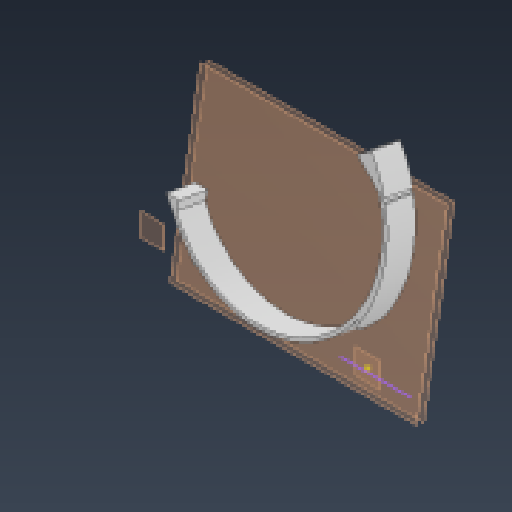
# Autodesk Inventor part: thigh_strap_03
Saved by Autodesk Inventor 2025.2 (Build 292293000, 293)
## iProperties
Created: 2025-03-07
Part Number: thigh_strap_03
Material: Generic
Document SubType Name: Modeling
Designer: email
Density: 1 g/cm^3
Appearance: Default
Author: email
Autodesk Inventor part; units mm, degrees
ref_plane "YZ Plane" through (0, 0, 0) normal (1, 0, 0) x (0, 1, 0)
ref_plane "XZ Plane" through (0, 0, 0) normal (0, 1, 0) x (-1, 0, 0)
ref_plane "Work Plane1" through (27.2016, 137.7902, -207.6153) normal (0, 0, 1) x (1, 0, 0)
ref_plane "Work Plane2" through (-81.5141, 115.844, -101.5145) normal (0, 0, 1) x (1, 0, 0)
sketch "Sketch2" plane through (27.2016, 137.7902, -207.6153) normal (0, 0, 1) x (1, 0, 0)
  line L0 (-50.9279, -141.1381) -> (10.2073, -141.1381)
  point P0 (-27.2016, -137.7902)
  constraints: 2 end point, 1 horizontal
ref_plane "Work Plane4" through (-23.7263, -2.2452, -201.3618) normal (0, 0.1736482, 0.9848078) x (1, 0, 0)
ref_plane "Work Plane3" through (-23.7263, -3.3479, -207.6153) normal (0, 0.1736482, 0.9848078) x (1, 0, 0)
sketch "Sketch1" plane through (-81.5141, 95.2083, -218.5455) normal (0, 0.1736482, 0.9848078) x (1, 0, 0)
  line L0 (120.3524, 26.6103) -> (110.8538, 39.0511) projected
  line L1 (109.9403, 39.2699) -> (118.8077, 27.6558) projected
  line L2 (117.4827, 25.3957) -> (118.8077, 27.6558) projected
  line L3 (108.6153, 37.0098) -> (109.9403, 39.2699) projected
  line L4 (-70.1644, -17.8234) -> (-70.1644, -42.3865) projected
  line L5 (-67.5144, -23.0328) -> (-67.5144, -49.6797) projected
  line L6 (-7.2549, -88.8185) -> (-7.2549, -90.7022)
  line L7 (88.6474, -22.0445) -> (90.1001, -24.6815)
  arc A0 (90.1001, -24.6815) -> (85.4909, 74.1551) centre (-2.6058, 20.521) ccw
  line L8 (68.6883, 59.486) -> (92.8567, 47.8109)
  ellipse E0 centre (117.3159, 24.5297) end of major axis (77.6327, 47.7943) minor radius 6.9177 (109.5288, 36.791) -> (89.1504, 46.193) ccw projected
  ellipse E1 centre (118.6409, 26.7898) end of major axis (80.226, 49.3108) minor radius 6.6966 (109.9403, 39.2699) -> (91.8991, 47.566) ccw projected
  line L9 (120.3524, 26.6103) -> (110.8538, 39.0511) projected
  line L10 (120.3524, 26.6103) -> (110.8538, 39.0511) projected
  line L11 (-70.1644, -47.9895) -> (-70.1644, -41.1809) projected
  line L12 (-78.1686, -54.9211) -> (-78.1686, -34.8) projected
  line L13 (-78.1686, -34.8) -> (-78.1686, -33.261) projected
  ellipse E2 centre (-68.1686, -34.8) end of major axis (-78.1686, -34.8) minor radius 8.1116 (-75.6686, -29.4347) -> (-78.1686, -34.8) ccw projected
  line L14 (-78.1686, -54.9211) -> (-78.1686, -34.8) projected
  line L15 (-77.6379, -18.1276) -> (-66.4488, -18.1276)
  line L16 (-66.4488, -18.1276) -> (-58.9889, -34.0305)
  arc A1 (-77.6379, -18.1276) -> (-51.8229, -55.9602) centre (98.8915, 74.6035) ccw
  line L17 (-51.8229, -55.9602) -> (-49.6664, -53.6662)
  ellipse E3 centre (43.7773, 28.2672) end of major axis (9.3333, 77.3077) minor radius 54.627 (86.8491, 61.886) -> (73.2137, 75.1203) ccw projected
  ellipse E4 centre (87.3016, 57.9812) end of major axis (48.0133, 78.9413) minor radius 0.2829 (58.2062, 73.2871) -> (75.8706, 63.7724) ccw projected
  ellipse E5 centre (86.0543, 55.6432) end of major axis (46.766, 76.6033) minor radius 0.2829 (56.9589, 70.9491) -> (74.6233, 61.4344) ccw projected
  ellipse E6 centre (-82.1686, -42.8548) end of major axis (-78.1686, -42.8548) minor radius 0.6946 (-78.1686, -42.8548) -> (-82.1686, -42.1602) ccw projected
  line L18 (85.4909, 74.1551) -> (63.6157, 67.3502)
  arc A2 (-66.1246, -22.0445) -> (76.0856, 61.886) centre (8.3655, 14.1852) ccw
  arc A3 (-70.1644, -30.1049) -> (79.8851, 69.6106) centre (7.0855, 16.4044) ccw
  line L19 (63.6157, 67.3502) -> (68.6883, 59.486)
  point P0 (81.5141, -131.7119)
  point P1 (-70.1644, -31.1405)
  point P2 (97.5203, 45.2683)
  point P3 (-67.5144, -35.2635)
  point P4 (96.3482, 45.7746)
  point P5 (98.1827, 42.4146)
  point P6 (110.3672, 38.7108)
  point P7 (-70.1644, -18.1276)
  point P8 (81.3429, 53.3729)
  point P9 (-67.5144, -34.2466)
  constraints: 16 end point, 11 point on circle, 4 centre point, 2 midpoint, 1 horizontal, 12 other
extrude "Extrusion1" add sketch "Sketch1" along normal blind 25.4 contours E0 A3 E3 L18 A0 | A0 L7 A3 E0 | A3 L4 L15 L16 A2 L8 | L8 L19 L18 E3 A3 | L17 A1 L5 A3 | L4 A1 L15
fillet "Fillet1" radius 12.7 4 edges at (7.8596, 76.6109, -189.4744) (7.8596, 72.2002, -214.4886) (-132.2588, 41.2279, -209.0273) (-132.2588, 45.6386, -184.0132)
body "Solid1"
